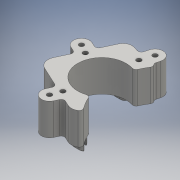
# Autodesk Inventor part: Adapter
Saved by Autodesk Inventor 2016 SP1 (Build 200210100, 210)
## iProperties
Created: 2015-11-17
Part Number: Adapter
Material: Generic
Document SubType Name: Modeling
Designer: PowerStation9000
Density: 1 g/cm^3
Appearance: Default
Author: PowerStation9000
Autodesk Inventor part; units mm, degrees
ref_plane "YZ Plane" through (0, 0, 0) normal (1, 0, 0) x (0, 1, 0)
ref_plane "XZ Plane" through (0, 0, 0) normal (0, 1, 0) x (-1, 0, 0)
ref_plane "XY Plane" through (0, 0, 0) normal (0, 0, 1) x (1, 0, 0)
sketch "Sketch1" plane through (0, 0, 0) normal (0, 0, 1) x (1, 0, 0)
  line L0 (-40.553928, 54.635427) -> (-37.554871, 54.635427)
  arc A0 (-40.553928, 61.835427) -> (-40.553928, 54.635427) centre (-40.553928, 58.235427) ccw
  line L1 (-40.553928, 61.835427) -> (-37.554871, 61.835427)
  arc A1 (-37.554871, 54.635427) -> (-37.554871, 61.835427) centre (-37.554871, 58.235427) ccw
  line L2 (-12.926163, 41.779167) -> (-9.925315, 41.779167) construction
  arc A2 (-12.926163, 48.979167) -> (-12.926163, 41.779167) centre (-12.926163, 45.379167) ccw construction
  line L3 (-12.926163, 48.979167) -> (-9.925315, 48.979167) construction
  arc A3 (-9.925315, 41.779167) -> (-9.925315, 48.979167) centre (-9.925315, 45.379167) ccw construction
  line L4 (-25.807813, 14.143602) -> (-22.823852, 14.143602)
  arc A4 (-25.807813, 21.343602) -> (-25.807813, 14.143602) centre (-25.807813, 17.743602) ccw construction
  line L5 (-25.807813, 21.343602) -> (-22.823852, 21.343602)
  arc A5 (-22.823852, 14.143602) -> (-22.823852, 21.343602) centre (-22.823852, 17.743602) ccw construction
  circle A6 centre (-31.685116, 37.989514) radius 15.19697 construction
  line L6 (-53.420483, 34.199862) -> (-50.436522, 34.199862) construction
  arc A7 (-50.436522, 26.999862) -> (-50.436522, 34.199862) centre (-50.436522, 30.599862) ccw construction
  line L7 (-50.436522, 26.999862) -> (-53.420483, 26.999862) construction
  arc A8 (-53.420483, 34.199862) -> (-53.420483, 26.999862) centre (-53.420483, 30.599862) ccw construction
  line L8 (-54.608076, 24.844676) -> (-41.009738, 18.513388)
  arc A9 (-26.995406, 11.988416) -> (-18.555169, 15.075824) centre (-24.315833, 17.743602) ccw construction
  line L9 (-18.555169, 15.075824) -> (-13.171982, 26.7) construction
  line L10 (-13.171982, 26.7) -> (-2.677813, 26.7) construction
  line L11 (-2.677813, 26.7) -> (-2.677813, 12.095348) construction
  line L12 (-2.677813, 12.095348) -> (21.322187, 12.095348) construction
  line L13 (21.322187, 12.095348) -> (21.322187, 34.85) construction
  arc A10 (21.322187, 41.15) -> (21.322187, 34.85) centre (10.522187, 38) ccw construction
  line L14 (21.322187, 41.15) -> (21.322187, 53) construction
  arc A11 (21.322187, 53) -> (15.322187, 59) centre (15.322187, 53) ccw construction
  line L15 (15.322187, 59) -> (0.20824, 59) construction
  arc A12 (-37.708705, 64.43957) -> (-32.903092, 63.055711) centre (-1.734787, 180.327275) ccw construction
  arc A13 (-37.708705, 64.43957) -> (-44.809013, 60.916229) centre (-39.0544, 58.235427) ccw construction
  line L16 (-44.809013, 60.916229) -> (-49.134667, 51.630775)
  arc A14 (-57.683116, 33.280665) -> (-54.608076, 24.844676) centre (-51.928503, 30.599862) ccw construction
  arc A15 (43.876221, 52.76945) -> (43.698618, 53.16419) centre (10.522187, 38) ccw construction
  circle A16 centre (10.522187, 38) radius 36.477778 construction
  arc A17 (-25.387924, 51.820396) -> (-25.381053, 24.161764) centre (-31.685116, 37.989514) ccw
  circle A18 centre (10.522187, 38) radius 38.477778
  arc A19 (-37.708705, 64.43957) -> (-20.708022, 60.476954) centre (-1.734787, 180.327275) ccw
  arc A20 (-37.708705, 64.43957) -> (-44.809013, 60.916229) centre (-39.411321, 58.954701) ccw
  arc A21 (-57.683116, 33.280665) -> (-54.608076, 24.844676) centre (-51.928503, 30.599862) ccw
  arc A22 (-26.995406, 11.988416) -> (-19.366583, 13.767773) centre (-24.315833, 17.743602) ccw
  circle A23 centre (-53.420483, 30.599862) radius 3.6
  circle A24 centre (-50.436522, 30.599862) radius 3.6
  circle A25 centre (-25.807813, 17.743602) radius 3.6
  arc A26 (-24.057995, 21.125449) -> (-20.391476, 15.089634) centre (-22.823852, 17.743602) ccw
  circle A27 centre (-38.587388, 11.870179) radius 2.25 construction
  circle A28 centre (-26.780732, 66.593373) radius 2.25 construction
  circle A29 centre (-55.778393, 49.209844) radius 2.25 construction
  line L17 (-53.666996, 53.742173) -> (-49.134667, 51.630775) construction
  arc A30 (-53.666996, 53.742173) -> (-57.889791, 44.677516) centre (-55.778393, 49.209844) ccw construction
  line L18 (-53.357462, 42.566119) -> (-57.889791, 44.677516) construction
  line L19 (-53.357462, 42.566119) -> (-57.683116, 33.280665)
  line L20 (-43.120167, 13.980608) -> (-41.009738, 18.513388) construction
  arc A31 (-43.120167, 13.980608) -> (-34.054609, 9.75975) centre (-38.587388, 11.870179) ccw construction
  line L21 (-31.944179, 14.292529) -> (-34.054609, 9.75975) construction
  line L22 (-31.944179, 14.292529) -> (-26.995406, 11.988416)
  arc A32 (-23.131901, 60.885881) -> (0.20824, 59) centre (-1.734787, 180.327275) ccw
  line L23 (-21.95062, 65.301083) -> (-23.131901, 60.885881) construction
  arc A33 (-21.95062, 65.301083) -> (-31.610845, 67.885663) centre (-26.780732, 66.593373) ccw construction
  line L24 (-32.903092, 63.055711) -> (-31.610845, 67.885663) construction
  line L25 (-49.134667, 51.630775) -> (-53.357462, 42.566119)
  line L26 (-41.009738, 18.513388) -> (-31.944179, 14.292529)
  point P0 (0, 0)
  dimension "d0" = 2
  constraints: 19 point on circle, 10 centre point, 7 concentric, 6 coincident, 4 end point, 3 tangent, 1 collinear, 3 other
extrude "Extrusion1" add sketch "Sketch1" along normal blind 20 contours A0 L1 A1 L0 | A25 A26 L4 | L4 A26 A18 A22 L22 L26 L8 A21 L19 L25 L16 A20 A19 A17 L5 A25 | A25 A26 | A26 A25 A18 | L5 A18 A26 A25 | A26 A25 A18 | A26 A18 A25 | A18 A25 | A23 A24 | A23 A24 | A24 A23 picked at (-23.00558, 19.443605)
sketch "Sketch3" plane through (0, 0, 0) normal (0, 0, -1) x (-1, 0, 0)
  arc A0 (40.553928, 54.635427) -> (40.553928, 61.835427) centre (40.553928, 58.235427) ccw construction
  line L0 (40.553928, 54.635427) -> (37.554871, 54.635427) construction
  arc A1 (37.554871, 61.835427) -> (37.554871, 54.635427) centre (37.554871, 58.235427) ccw construction
  line L1 (37.554871, 61.835427) -> (40.553928, 61.835427) construction
  line L2 (40.553928, 56.235427) -> (37.554871, 56.235427)
  arc A2 (40.553928, 56.235427) -> (40.553928, 60.235427) centre (40.553928, 58.235427) ccw
  line L3 (40.553928, 60.235427) -> (37.554871, 60.235427)
  arc A3 (37.554871, 60.235427) -> (37.554871, 56.235427) centre (37.554871, 58.235427) ccw
  arc A4 (50.436522, 32.599862) -> (50.436522, 28.599862) centre (50.436522, 30.599862) ccw
  line L4 (53.420483, 28.599862) -> (50.436522, 28.599862)
  arc A5 (53.420483, 28.599862) -> (53.420483, 32.599862) centre (53.420483, 30.599862) ccw
  line L5 (50.436522, 32.599862) -> (53.420483, 32.599862)
  arc A6 (53.420483, 26.999862) -> (53.420483, 34.199862) centre (53.420483, 30.599862) ccw construction
  line L6 (50.436522, 26.999862) -> (53.420483, 26.999862) construction
  arc A7 (50.436522, 34.199862) -> (50.436522, 26.999862) centre (50.436522, 30.599862) ccw construction
  line L7 (53.420483, 34.199862) -> (50.436522, 34.199862) construction
  arc A8 (25.807813, 14.143602) -> (25.807813, 21.343602) centre (25.807813, 17.743602) ccw construction
  line L8 (25.807813, 14.143602) -> (22.823852, 14.143602) construction
  arc A9 (22.823852, 21.343602) -> (22.823852, 14.143602) centre (22.823852, 17.743602) ccw construction
  line L9 (22.823852, 21.343602) -> (25.807813, 21.343602) construction
  line L10 (25.807813, 15.743602) -> (22.823852, 15.743602)
  arc A10 (25.807813, 15.743602) -> (25.807813, 19.743602) centre (25.807813, 17.743602) ccw
  line L11 (25.807813, 19.743602) -> (22.823852, 19.743602)
  arc A11 (22.823852, 19.743602) -> (22.823852, 15.743602) centre (22.823852, 17.743602) ccw
  line L12 (22.823852, 14.643602) -> (25.807813, 14.643602)
  arc A12 (25.807813, 14.643602) -> (25.807813, 20.843602) centre (25.807813, 17.743602) ccw
  line L13 (25.807813, 20.843602) -> (22.823852, 20.843602)
  arc A13 (22.823852, 20.843602) -> (22.823852, 14.643602) centre (22.823852, 17.743602) ccw
  line L14 (50.436522, 27.499862) -> (53.420483, 27.499862)
  arc A14 (53.420483, 27.499862) -> (53.420483, 33.699862) centre (53.420483, 30.599862) ccw
  line L15 (53.420483, 33.699862) -> (50.436522, 33.699862)
  arc A15 (50.436522, 33.699862) -> (50.436522, 27.499862) centre (50.436522, 30.599862) ccw
  line L16 (37.554871, 55.135427) -> (40.553928, 55.135427)
  arc A16 (40.553928, 55.135427) -> (40.553928, 61.335427) centre (40.553928, 58.235427) ccw
  line L17 (40.553928, 61.335427) -> (37.554871, 61.335427)
  arc A17 (37.554871, 61.335427) -> (37.554871, 55.135427) centre (37.554871, 58.235427) ccw
  point P0 (0, 0)
  dimension "d7" = 0.5
  dimension "d8" = 0.5
  dimension "d9" = 0.5
  constraints: 12 end point, 12 point on circle, 6 centre point, 9 other
  measures "d7" radial gap between concentric circles of A9 A13
  measures "d8" radial gap between concentric circles of A7 A15
  measures "d9" radial gap between concentric circles of A1 A17
extrude "Extrusion3" add sketch "Sketch3" along normal blind 4
sketch "Sketch4" plane through (0, 0, 20) normal (0, 0, 1) x (1, 0, 0)
  arc A0 (-25.381053, 24.161764) -> (-23.893494, 20.792435) centre (10.522187, 38) ccw construction
  circle A1 centre (10.522187, 38) radius 38.477778
  point P0 (0, 0)
  point P1 (-24.1636, 21.343602)
  point P2 (-24.057995, 21.125449)
  constraints: 1 centre point, 1 coincident, 1 concentric
extrude "Extrusion4" cut sketch "Sketch4" against normal blind 46.5
sketch "Sketch6" plane through (0, 0, 0) normal (0, 0, -1) x (-1, 0, 0)
  circle A0 centre (38.587388, 11.870179) radius 2.25 construction
  circle A1 centre (26.780732, 66.593373) radius 2.25 construction
  circle A2 centre (55.778393, 49.209844) radius 2.25 construction
  circle A3 centre (31.685116, 37.989514) radius 15.19697 construction
  line L0 (25.807813, 15.743602) -> (22.823852, 15.743602) construction
  arc A4 (22.823852, 19.743602) -> (22.823852, 15.743602) centre (22.823852, 17.743602) ccw construction
  line L1 (22.823852, 19.743602) -> (25.807813, 19.743602) construction
  arc A5 (25.807813, 15.743602) -> (25.807813, 19.743602) centre (25.807813, 17.743602) ccw construction
  line L2 (12.926163, 43.379167) -> (9.925315, 43.379167) construction
  arc A6 (9.925315, 47.379167) -> (9.925315, 43.379167) centre (9.925315, 45.379167) ccw construction
  line L3 (9.925315, 47.379167) -> (12.926163, 47.379167) construction
  arc A7 (12.926163, 43.379167) -> (12.926163, 47.379167) centre (12.926163, 45.379167) ccw construction
  line L4 (40.553928, 56.235427) -> (37.554871, 56.235427) construction
  arc A8 (37.554871, 60.235427) -> (37.554871, 56.235427) centre (37.554871, 58.235427) ccw construction
  line L5 (37.554871, 60.235427) -> (40.553928, 60.235427) construction
  arc A9 (40.553928, 56.235427) -> (40.553928, 60.235427) centre (40.553928, 58.235427) ccw construction
  arc A10 (53.420483, 28.599862) -> (53.420483, 32.599862) centre (53.420483, 30.599862) ccw construction
  line L6 (50.436522, 28.599862) -> (53.420483, 28.599862) construction
  arc A11 (50.436522, 32.599862) -> (50.436522, 28.599862) centre (50.436522, 30.599862) ccw construction
  line L7 (53.420483, 32.599862) -> (50.436522, 32.599862) construction
  arc A12 (2.677813, 58.988107) -> (23.131901, 60.885881) centre (1.734787, 180.327275) ccw construction
  line L8 (2.677813, 58.988107) -> (2.677813, 55.885049) construction
  line L9 (2.677813, 55.885049) -> (13.427813, 55.885049) construction
  line L10 (13.427813, 55.885049) -> (13.427813, 53.714951) construction
  line L11 (13.427813, 53.714951) -> (2.677813, 53.714951) construction
  line L12 (2.677813, 53.714951) -> (2.677813, 26.7) construction
  line L13 (2.677813, 26.7) -> (13.171982, 26.7) construction
  line L14 (13.171982, 26.7) -> (18.555169, 15.075824) construction
  arc A13 (18.555169, 15.075824) -> (26.995406, 11.988416) centre (24.315833, 17.743602) ccw construction
  line L15 (31.944179, 14.292529) -> (26.995406, 11.988416) construction
  line L16 (31.944179, 14.292529) -> (34.054609, 9.75975) construction
  arc A14 (34.054609, 9.75975) -> (43.120167, 13.980608) centre (38.587388, 11.870179) ccw construction
  line L17 (43.120167, 13.980608) -> (41.009738, 18.513388) construction
  line L18 (54.608076, 24.844676) -> (41.009738, 18.513388) construction
  arc A15 (54.608076, 24.844676) -> (57.683116, 33.280665) centre (51.928503, 30.599862) ccw construction
  line L19 (53.357462, 42.566119) -> (57.683116, 33.280665) construction
  line L20 (57.889791, 44.677516) -> (53.357462, 42.566119) construction
  arc A16 (57.889791, 44.677516) -> (53.666996, 53.742173) centre (55.778393, 49.209844) ccw construction
  line L21 (49.134667, 51.630775) -> (53.666996, 53.742173) construction
  line L22 (44.809013, 60.916229) -> (49.134667, 51.630775) construction
  arc A17 (44.809013, 60.916229) -> (37.708705, 64.43957) centre (39.0544, 58.235427) ccw construction
  arc A18 (32.903092, 63.055711) -> (37.708705, 64.43957) centre (1.734787, 180.327275) ccw construction
  line L23 (32.903092, 63.055711) -> (31.610845, 67.885663) construction
  arc A19 (31.610845, 67.885663) -> (21.95062, 65.301083) centre (26.780732, 66.593373) ccw construction
  line L24 (21.95062, 65.301083) -> (23.131901, 60.885881) construction
  arc A20 (57.889791, 44.677516) -> (53.666996, 53.742173) centre (55.778393, 49.209844) ccw
  line L25 (57.889791, 44.677516) -> (53.357462, 42.566119)
  line L26 (53.357462, 42.566119) -> (49.134667, 51.630775)
  line L27 (44.809013, 60.916229) -> (57.683116, 33.280665)
  line L28 (49.134667, 51.630775) -> (53.666996, 53.742173)
  circle A21 centre (55.778393, 49.209844) radius 1.5
  circle A22 centre (26.780732, 66.593373) radius 1.5
  line L29 (31.610845, 67.885663) -> (32.903092, 63.055711)
  line L30 (23.131901, 60.885881) -> (21.95062, 65.301083)
  arc A23 (23.131901, 60.885881) -> (32.903092, 63.055711) centre (1.734787, 180.327275) ccw
  arc A24 (20.708022, 60.476954) -> (37.708705, 64.43957) centre (1.734787, 180.327275) ccw construction
  arc A25 (31.610845, 67.885663) -> (21.95062, 65.301083) centre (26.780732, 66.593373) ccw
  arc A26 (34.054609, 9.75975) -> (43.120167, 13.980608) centre (38.587388, 11.870179) ccw
  line L31 (43.120167, 13.980608) -> (41.009738, 18.513388)
  line L32 (41.009738, 18.513388) -> (31.944179, 14.292529)
  line L33 (54.608076, 24.844676) -> (26.995406, 11.988416)
  line L34 (31.944179, 14.292529) -> (34.054609, 9.75975)
  circle A27 centre (38.587388, 11.870179) radius 1.5
  point P0 (0, 0)
  dimension "d14" = 3
  dimension "d16" = 3
  dimension "d17" = 3
  constraints: 16 end point, 8 point on circle, 7 centre point, 6 coincident, 6 tangent, 5 collinear, 4 point on line, 2 concentric
  measures "d14" diameter of A21
  measures "d16" diameter of A22
  measures "d17" diameter of A27
extrude "Extruder montering" add sketch "Sketch6" against normal up to surface (20 mm away)
fillet "Fillet1" radius 2 10 edges at (-53.3575, 42.5661, 10) (-49.1347, 51.6308, 10) (-32.9031, 63.0557, 10) (-23.1319, 60.8859, 10) (-20.708, 60.477, 10) (-25.3879, 51.8204, 10) (-25.3811, 24.1618, 10) (-19.3666, 13.7678, 10) (-31.9442, 14.2925, 10) (-41.0097, 18.5134, 10)
sketch "Sketch7" plane through (0, 0, 0) normal (0, 0, -1) x (-1, 0, 0)
  circle A0 centre (26.780732, 66.593373) radius 1.5 construction
  arc A1 (22.109856, 61.14218) -> (21.902022, 58.717386) centre (23.587369, 59.794235) ccw construction
  arc A2 (22.109856, 61.14218) -> (22.564388, 63.00704) centre (20.632343, 62.490124) ccw construction
  line L0 (21.95062, 65.301083) -> (22.564388, 63.00704) construction
  arc A3 (31.610845, 67.885663) -> (21.95062, 65.301083) centre (26.780732, 66.593373) ccw construction
  line L1 (32.382712, 65.000702) -> (31.610845, 67.885663) construction
  arc A4 (32.382712, 65.000702) -> (34.860746, 63.593587) centre (34.314757, 65.517618) ccw construction
  arc A5 (34.860746, 63.593587) -> (37.708705, 64.43957) centre (1.734787, 180.327275) ccw construction
  arc A6 (44.809013, 60.916229) -> (37.708705, 64.43957) centre (39.411321, 58.954701) ccw construction
  line L2 (44.809013, 60.916229) -> (48.290108, 53.443707) construction
  arc A7 (48.290108, 53.443707) -> (50.947599, 52.475334) centre (50.10304, 54.288266) ccw construction
  line L3 (53.666996, 53.742173) -> (50.947599, 52.475334) construction
  arc A8 (53.666996, 53.742173) -> (57.889791, 44.677516) centre (55.778393, 49.209844) ccw construction
  line L4 (55.170394, 43.410678) -> (57.889791, 44.677516) construction
  arc A9 (54.608076, 24.844676) -> (57.683116, 33.280665) centre (51.928503, 30.599862) ccw construction
  line L5 (54.608076, 24.844676) -> (42.82285, 19.357559) construction
  arc A10 (42.82285, 19.357559) -> (41.85391, 16.700276) centre (43.667021, 17.544448) ccw construction
  line L6 (43.120167, 13.980608) -> (41.85391, 16.700276) construction
  arc A11 (43.120167, 13.980608) -> (34.054609, 9.75975) centre (38.587388, 11.870179) ccw construction
  line L7 (32.788351, 12.479417) -> (34.054609, 9.75975) construction
  arc A12 (21.055092, 12.296598) -> (26.995406, 11.988416) centre (24.315833, 17.743602) ccw construction
  arc A13 (20.47137, 15.197832) -> (21.055092, 12.296598) centre (22.082355, 14.01262) ccw construction
  arc A14 (20.47137, 15.197832) -> (24.655132, 22.408476) centre (-10.522187, 38) ccw construction
  arc A15 (27.088517, 23.504378) -> (24.655132, 22.408476) centre (26.483581, 21.598059) ccw construction
  arc A16 (27.088517, 23.504378) -> (27.095715, 52.476933) centre (31.685116, 37.989514) ccw construction
  arc A17 (24.662875, 53.574044) -> (27.095715, 52.476933) centre (26.491726, 54.383552) ccw construction
  arc A18 (24.662875, 53.574044) -> (21.902022, 58.717386) centre (-10.522187, 38) ccw construction
  circle A19 centre (36.287315, 17.981062) radius 4.5
  circle A20 centre (50.10304, 45.957908) radius 4.5
  circle A21 centre (29.359507, 58.954701) radius 4.5
  line L8 (54.202021, 40.753187) -> (57.683116, 33.280665)
  line L9 (30.131068, 13.448357) -> (26.995406, 11.988416)
  arc A22 (55.170394, 43.410678) -> (54.202021, 40.753187) centre (56.014953, 41.597746) ccw
  arc A23 (32.788351, 12.479417) -> (30.131068, 13.448357) centre (30.975239, 11.635246) ccw
  point P0 (0, 0)
  dimension "d21" = 9
  dimension "d22" = 9
  dimension "d23" = 9
  constraints: 3 centre point
  measures "d21" diameter of A19
  measures "d22" diameter of A20
  measures "d23" diameter of A21
extrude "Extrusion7" cut sketch "Sketch7" against normal blind 16
sketch "Sketch8" plane through (-50.10304, 45.957908, 16) normal (0, 0, -1) x (-1, 0, 0)
  circle A0 centre (-13.815725, -27.976846) radius 4.5
  circle A1 centre (-20.743532, 12.996793) radius 4.5
  circle A2 centre (0, 0) radius 4.5
  circle A3 centre (-13.815725, -27.976846) radius 1.5
  circle A4 centre (0, 0) radius 1.5
  circle A5 centre (-20.743532, 12.996793) radius 1.5
  point P0 (-50.10304, -45.957908)
  dimension "d26" = 3
  dimension "d27" = 3
  dimension "d28" = 3
  constraints: 3 centre point, 3 coincident
  measures "d26" diameter of A3
  measures "d27" diameter of A4
  measures "d28" diameter of A5
extrude "Extrusion8" cut sketch "Sketch8" against normal up to surface (4 mm away) contours A3 | A4 | A5
chamfer "Chamfer1" distance 0.5 angle 45 12 edges at (-51.9285, 33.6999, -4) (-47.3365, 30.5999, -4) (-51.9285, 27.4999, -4) (-56.5205, 30.5999, -4) (-43.6539, 58.2354, -4) (-39.0544, 61.3354, -4) (-34.4549, 58.2354, -4) (-39.0544, 55.1354, -4) (-28.9078, 17.7436, -4) (-24.8634, 20.8436, -4) (-24.3158, 14.6436, -4) (-21.6743, 14.8646, -4)
chamfer "Chamfer2" distance 0.5 angle 45 3 edges at (-37.0874, 11.8702, 0) (-54.2784, 49.2098, 0) (-25.2807, 66.5934, 0)
equation "\"d27\" = d26"
equation "\"d28\" = d26"
body "Solid1"
